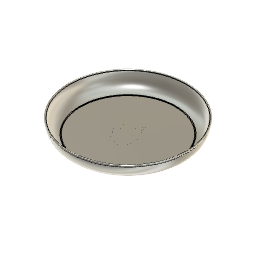
RFID ID-12LA Plate (Autodesk Fusion 360 design; units mm, degrees)
Autodesk Fusion 360 part; units mm, degrees
sketch "Sketch1" plane through (0, 0, 0) normal (0, 0, 1) x (1, 0, 0) in component "RFID Reader: ID-12LA"
  line L0 (12.75, -12.25) -> (-12.75, -12.25)
  line L1 (-12.75, -12.25) -> (-12.75, 12.25)
  line L2 (-12.75, 12.25) -> (12.75, 12.25)
  line L3 (12.75, 12.25) -> (12.75, -12.25)
  line L4 (12.75, -12.25) -> (-12.75, 12.25) construction
  line L5 (-12.75, -12.25) -> (12.75, 12.25) construction
  dimension "d6" = 25.5
  dimension "d7" = 24.5
  constraint horizontal L0
  constraint perpendicular L0 L1
  constraint parallel L0 L2
  constraint parallel L1 L3
  constraint coincident L4 origin
  constraint coincident L5 origin
  measures "d6" distance of L1.end L2.end
  measures "d7" distance of L0.end L1.end
extrude "Extrude1" add sketch "Sketch1" along normal blind 6 makes body 1 in component "RFID Reader: ID-12LA"
fillet "Fillet1" radius 1 8 edges at (12.75, -12.25, 3) (12.75, 0, 6) (0, -12.25, 6) (-12.75, -12.25, 3) (-12.75, 0, 6) (0, 12.25, 6) (12.75, 12.25, 3) (-12.75, 12.25, 3) on bodies 1 in component "RFID Reader: ID-12LA"
sketch "Scale's plate sketch." plane through (0, 0, 0) normal (0, 1, 0) x (1, 0, 0) in component "Plate"
  line L0 (66.5889, 0) -> (-82.2802, 0)
  line L1 (-82.2802, 0) -> (-82.2802, -21)
  line L2 (-82.2802, -21) -> (82.8198, -21)
  line L3 (82.8198, 0) -> (-82.2802, -21) construction
  line L4 (-82.2802, 0) -> (82.8198, -21) construction
  line L5 (1.75, 0) -> (22.5, 0)
  line L6 (0, 0) -> (0, -1.2)
  line L7 (0, -1.2) -> (66.4869, -1.2)
  line L8 (82.8198, -21) -> (81.6198, -21) construction
  arc A0 (81.6198, -21) -> (67.5901, -1.3232) centre (63.5877, -19.017) ccw
  arc A1 (82.8198, -21) -> (67.4732, -0.0788) centre (64.1431, -18.6109) ccw
  arc A2 (67.5901, -1.3232) -> (66.4869, -1.2) centre (66.4869, -6.2) ccw
  arc A3 (67.4732, -0.0788) -> (66.5889, 0) centre (66.5889, -5) ccw
  circle A4 centre (82.8198, -21) radius 1.2
  point P0 (0.2698, -10.5)
  dimension "d16" = 165.1
  dimension "d17" = 21
  dimension "d18" = 1.2
  dimension "d19" = 1.2
  dimension "d20" = 5
  dimension "d21" = 5
  constraint horizontal L0
  constraint perpendicular L0 L1
  constraint parallel L0 L2
  constraint coincident L3 P0
  constraint coincident L4 P0
  constraint collinear L0 L5
  constraint coincident L6.start origin
  constraint perpendicular L0 L6
  constraint perpendicular L6 L7
  constraint tangent A0 A1
  constraint tangent L7 A2
  constraint tangent A0 A2
  constraint tangent L0 A3
  constraint tangent A1 A3
  constraint coincident L2.end L4.end
  constraint coincident L8.end A4
  measures "d16" distance of L1.end L2.end
  measures "d17" distance of L0.end L1.end
  measures "d18" distance of L6.start L6.end
  measures "d19" distance of L2.end L8.end
  measures "d20" radius of A2
  measures "d21" radius of A3
revolve "Revolution of the scale's plate sketch." add sketch "Scale's plate sketch." angle 360 about axis through (0, 0, 1.75) along (0, 0, 1) separate body contours L0 L5 L6 L7 A0 A1 A2 A3 A4 | L2 A1 A4 | L2 A0 A1 A4 makes body 2 in component "Plate"
sketch "RFID mount area sketch." plane through (0, 0, 0) normal (0, 0, -1) x (1, 0, 0) in component "Plate"
  circle A0 centre (0, 0) radius 66.5889
  arc A1 (-12.75, -11.25) -> (-11.75, -12.25) centre (-11.75, -11.25) ccw
  line L0 (-11.75, -12.25) -> (11.75, -12.25)
  arc A2 (11.75, -12.25) -> (12.75, -11.25) centre (11.75, -11.25) ccw
  line L1 (12.75, -11.25) -> (12.75, 11.25)
  arc A3 (12.75, 11.25) -> (11.75, 12.25) centre (11.75, 11.25) ccw
  line L2 (11.75, 12.25) -> (-11.75, 12.25)
  arc A4 (-11.75, 12.25) -> (-12.75, 11.25) centre (-11.75, 11.25) ccw
  line L3 (-12.75, 11.25) -> (-12.75, -11.25)
  line L4 (11.75, 12.55) -> (-11.75, 12.55)
  arc A5 (-11.75, 12.55) -> (-13.05, 11.25) centre (-11.75, 11.25) ccw
  line L5 (-13.05, 11.25) -> (-13.05, -11.25)
  arc A6 (-13.05, -11.25) -> (-11.75, -12.55) centre (-11.75, -11.25) ccw
  line L6 (-11.75, -12.55) -> (11.75, -12.55)
  arc A7 (11.75, -12.55) -> (13.05, -11.25) centre (11.75, -11.25) ccw
  line L7 (13.05, -11.25) -> (13.05, 11.25)
  arc A8 (13.05, 11.25) -> (11.75, 12.55) centre (11.75, 11.25) ccw
  line L8 (11.75, 14.55) -> (-11.75, 14.55)
  arc A9 (-11.75, 14.55) -> (-15.05, 11.25) centre (-11.75, 11.25) ccw
  line L9 (-15.05, 11.25) -> (-15.05, -11.25)
  arc A10 (-15.05, -11.25) -> (-11.75, -14.55) centre (-11.75, -11.25) ccw
  line L10 (-11.75, -14.55) -> (11.75, -14.55)
  arc A11 (11.75, -14.55) -> (15.05, -11.25) centre (11.75, -11.25) ccw
  line L11 (15.05, -11.25) -> (15.05, 11.25)
  arc A12 (15.05, 11.25) -> (11.75, 14.55) centre (11.75, 11.25) ccw
  circle A13 centre (0, 20) radius 2.3
  line L12 (0, -1.75) -> (0, -22.5)
  line L13 (1.75, 0) -> (22.5, 0)
  circle A14 centre (0, -20) radius 2.3
  circle A15 centre (-18, 0) radius 1.5
  circle A16 centre (18, 0) radius 1.5
  circle A17 centre (0, 20) radius 4.3
  line L14 (0, 20) -> (4.3, 20) construction
  line L15 (0, 20) -> (-4.3, 20) construction
  line L16 (4.3, 20) -> (4.3, 14.55)
  line L17 (-4.3, 20) -> (-4.3, 14.55)
  circle A18 centre (-18, 0) radius 2.7
  line L18 (-18, 0) -> (-18, 2.7) construction
  line L19 (-18, 0) -> (-18, -2.7) construction
  line L20 (-18, -2.7) -> (-15.05, -2.7)
  line L21 (-18, 2.7) -> (-15.05, 2.7)
  line L22 (-4.3, -20) -> (-4.3, -14.55)
  circle A19 centre (0, -20) radius 4.3
  line L23 (4.3, -20) -> (4.3, -14.55)
  circle A20 centre (18, 0) radius 2.7
  line L24 (18, 2.7) -> (15.05, 2.7)
  line L25 (18, -2.7) -> (15.05, -2.7)
  dimension "d23" = 0.3
  dimension "d24" = 2.3
  dimension "d29" = 4.6
  dimension "d30" = 20
  dimension "d31" = 3
  dimension "d32" = 18
  dimension "d33" = 2
  dimension "d34" = 1.2
  constraint coincident A13.centre L12
  constraint symmetric A13 L13 A14
  constraint coincident L13 A15.centre
  constraint symmetric L12 A15 A16
  constraint coincident A13.centre A17.centre
  constraint coincident A17 L14.end
  constraint horizontal L14
  constraint coincident A17 L15.end
  constraint parallel L14 L15
  constraint coincident L8 L16.end
  constraint tangent A17 L16
  constraint coincident L8 L17.end
  constraint tangent A17 L17
  constraint coincident A15.centre A18.centre
  constraint coincident A18 L18.end
  constraint vertical L18
  constraint coincident A18 L19.end
  constraint parallel L18 L19
  constraint coincident L9 L20.end
  constraint tangent A18 L20
  constraint coincident L9 L21.end
  constraint tangent A18 L21
  constraint symmetric L13 A17 A19
  constraint symmetric L13 L14.end L23.start
  constraint symmetric L13 L15.end L22.start
  constraint symmetric L13 L16.end L23.end
  constraint symmetric L13 L17.end L22.end
  constraint symmetric L12 A18 A20
  constraint symmetric L12 L18.end L24.start
  constraint symmetric L12 L19.end L25.start
  constraint symmetric L12 L20.end L25.end
  constraint symmetric L12 L21.end L24.end
  measures "d29" diameter of A13
  measures "d30" distance of A0.centre A13.centre
  measures "d31" diameter of A15
  measures "d32" distance of L12 A15.centre
extrude "Extrude1'" add sketch "RFID mount area sketch." along normal blind 5 contours L4 A5 L5 A6 L6 L7 A8 L8 A9 L9 A10 L10 L11 A12 L12 L13 | L6 A7 L7 L10 A11 L11 L12 L13 | L10 L12 L22 A19 | L10 L12 A19 L23 | A19 | L11 L13 A20 L25 | L11 L13 A20 L24 | L13 A16 A20 | L13 A16 A20 | L9 A18 L20 L21 | A18 | L8 A17 L16 L17 | A17 bodies 2 in component "Plate"
component "RFID Reader: ID-12LA" placed x (1, 0, 0) y (0, 1, 0) z (0, 0, 1) at (0, 0, 0)
component "Plate" placed x (1, 0, 0) y (0, 1, 0) z (0, 0, 1) at (0, 0, 6.3)
equation "s_tolerance = 0.1 mm" comment "Small tolerance of the 3D printer."
equation "b_tolerance = 0.3 mm" comment "Big tolerance of the 3D printer."
equation "rfid_width = 24.5 mm" comment "Width of the rfid reader."
equation "rfid_length = 25.5 mm" comment "Length of the rfid reader."
equation "rfid_height = 6 mm" comment "Height of the rfid reader."
equation "d6 = rfid_length"
equation "d7 = rfid_width"
equation "d8 = rfid_height"
equation "rfid_fillet = 1 mm" comment "Fillet of the rfid top edges."
equation "d12 = rfid_fillet"
equation "plate_height = 21 mm" comment "Height of the scale's plates."
equation "plate_diam = 6.5 in" comment "Diameter of the scale's plates."
equation "plate_thick = 1.2 mm" comment "Thickness of the scale's plate."
equation "d16 = plate_diam"
equation "d17 = plate_height"
equation "d18 = plate_thick"
equation "d19 = plate_thick"
equation "d23 = b_tolerance"
equation "d24 = b_tolerance + plate_rfid_perimeter_offset"
equation "plate_rfid_perimeter_offset = 2 mm" comment "Offset of the perimeter surrounding the rfid beneath the plate."
equation "plate_rfid_guide_diam = 3 mm" comment "Diameter of the guide pins for the mounting of the rfid to the plate."
equation "m3_threaded_insert_diam = 4.6 mm" comment "Diameter of the M3 threaded inserts to be used to mount the rfids to the plate."
equation "plate_rfid_mheight = 5 mm" comment "Height of the mount area for the rfid underneath the plate."
equation "d29 = m3_threaded_insert_diam"
equation "d31 = plate_rfid_guide_diam"
equation "d35 = plate_rfid_mheight"
